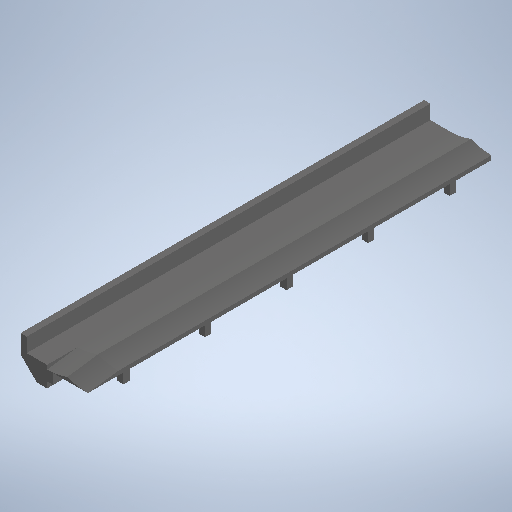
# Autodesk Inventor part: front_rail
Saved by Autodesk Inventor 2026.1 (Build 301233020, 233B)
## iProperties
Created: 2025-09-28
Part Number: front_rail
Material: 一般
Document SubType Name: Modeling
Designer: hibik
Density: 1 g/cm^3
Appearance: 既定
Author: hibik
Autodesk Inventor part; units mm, degrees
ref_plane "YZ Plane" through (0, 0, 0) normal (1, 0, 0) x (0, 1, 0)
ref_plane "XZ Plane" through (0, 0, 0) normal (0, 1, 0) x (-1, 0, 0)
ref_plane "XY Plane" through (0, 0, 0) normal (0, 0, 1) x (1, 0, 0)
sketch "スケッチ1" plane through (0, 0, 0) normal (0, 1, 0) x (-1, 0, 0)
  line L0 (0, 99) -> (20, 99)
  line L1 (20, 99) -> (20, -99)
  line L2 (20, -99) -> (0, -99)
  line L3 (0, -99) -> (0, 99)
  line L4 (20, -99) -> (20, -109)
  line L5 (20, -109) -> (9, -109)
  line L6 (9, -109) -> (11, -99)
  line L7 (10.5, 99) -> (8.5, 88.5)
  line L8 (8.5, 88.5) -> (20, 88.5)
  point P0 (0, 0)
  point P1 (0, 0)
  point P2 (10, -99)
  point P3 (10, 99)
  dimension "d0" = 198
  dimension "d1" = 20
  dimension "d4" = 10
  dimension "d5" = 1
  dimension "d6" = 1
  dimension "d7" = 10.5
  dimension "d8" = 1.5
  dimension "d9" = 0.5
  constraints: 18 end point, 3 midpoint, 3 perpendicular, 3 point on line, 2 parallel, 1 coincident, 1 horizontal, 1 vertical
  measures "d0" distance of L0.end L1.end
  measures "d1" distance of L0.start L0.end
  measures "d4" distance of L1.end L4.end
  measures "d5" distance of point (10, -99) L6.end
  measures "d6" horizontal distance of point (10, -99) L5.end
  measures "d7" distance between parallel lines of L0 L8
  measures "d8" horizontal distance of point (10, 99) L7.end
  measures "d9" distance of point (10, 99) L7.start
extrude "押し出し1" add sketch "スケッチ1" along normal blind 5.5 contours L0 L7 L8 L1 L2 L3 | L2 L4 L5 L6
sketch "スケッチ2" plane through (0, 5.5, 0) normal (0, 1, 0) x (1, 0, 0)
  line L0 (-20, 109) -> (-20, -88.5) projected
  line L1 (-20, -1.5) -> (-17, -1.5)
  line L2 (-17, -1.5) -> (-17, 1.5)
  line L3 (-17, 1.5) -> (-20, 1.5)
  line L4 (-20, 1.5) -> (-20, -1.5)
  line L5 (0, -99) -> (0, 99) projected
  line L6 (0, -1.5) -> (-3, -1.5)
  line L7 (-3, -1.5) -> (-3, 1.5)
  line L8 (-3, 1.5) -> (0, 1.5)
  line L9 (0, 1.5) -> (0, -1.5)
  point P0 (0, 0)
  point P1 (-17, 0)
  point P2 (0, 0)
  point P3 (0, 1.5)
  dimension "d10" = 3
  dimension "d11" = 3
  constraints: 16 end point, 4 parallel, 4 point on line, 2 horizontal, 2 midpoint, 2 perpendicular, 1 collinear, 1 horizontal alignment
  measures "d10" distance of L1.start L1.end
  measures "d11" distance of L1.end L2.end
extrude "押し出し2" cut sketch "スケッチ2" against normal through all
pattern_linear "矩形状パターン1" count 3 spacing 40 along (0, 0, -1) count 3 spacing 40 along (0, 0, 1) of "押し出し2"
sketch "スケッチ3" plane through (0, 5.5, 0) normal (0, 1, 0) x (1, 0, 0)
  line L0 (-20, -88.5) -> (-8.5, -88.5) projected
  line L1 (-20, -99) -> (0, -99)
  line L2 (0, -99) -> (0, 99)
  line L3 (0, 99) -> (-20.1365, 99)
  line L4 (-20, 109) -> (-20, -88.4991)
  line L5 (-20, -38.5) -> (-17, -38.5) projected
  line L6 (-17, -38.5) -> (-17, -41.5) projected
  line L7 (-17, -41.5) -> (-20, -41.5) projected
  line L8 (-20, -41.5) -> (-20, -78.5) projected
  line L9 (-20, -78.5) -> (-17, -78.5) projected
  line L10 (-17, -78.5) -> (-17, -81.5) projected
  line L11 (-17, -81.5) -> (-20, -81.5) projected
  line L12 (-20, -81.5) -> (-20, -88.5) projected
  line L13 (-20, -88.5) -> (-8.5, -88.5) projected
  line L14 (-8.5, -88.5) -> (-10.5, -99) projected
  line L15 (-10.5, -99) -> (0, -99) projected
  line L16 (0, -99) -> (0, -81.5) projected
  line L17 (0, -81.5) -> (-3, -81.5) projected
  line L18 (-3, -81.5) -> (-3, -78.5) projected
  line L19 (-3, -78.5) -> (0, -78.5) projected
  line L20 (0, -78.5) -> (0, -41.5) projected
  line L21 (0, -41.5) -> (-3, -41.5) projected
  line L22 (-3, -41.5) -> (-3, -38.5) projected
  line L23 (-3, -38.5) -> (0, -38.5) projected
  line L24 (0, -38.5) -> (0, -1.5) projected
  line L25 (0, -1.5) -> (-3, -1.5) projected
  line L26 (-3, -1.5) -> (-3, 1.5) projected
  line L27 (-3, 1.5) -> (0, 1.5) projected
  line L28 (0, 1.5) -> (0, 38.5) projected
  line L29 (0, 38.5) -> (-3, 38.5) projected
  line L30 (-3, 38.5) -> (-3, 41.5) projected
  line L31 (-3, 41.5) -> (0, 41.5) projected
  line L32 (0, 41.5) -> (0, 78.5) projected
  line L33 (0, 78.5) -> (-3, 78.5) projected
  line L34 (-3, 78.5) -> (-3, 81.5) projected
  line L35 (-3, 81.5) -> (0, 81.5) projected
  line L36 (0, 81.5) -> (0, 99) projected
  line L37 (0, 99) -> (-11, 99) projected
  line L38 (-11, 99) -> (-9, 109) projected
  line L39 (-9, 109) -> (-20, 109) projected
  line L40 (-20, 109) -> (-20, 81.5) projected
  line L41 (-20, 81.5) -> (-17, 81.5) projected
  line L42 (-17, 81.5) -> (-17, 78.5) projected
  line L43 (-17, 78.5) -> (-20, 78.5) projected
  line L44 (-20, 78.5) -> (-20, 41.5) projected
  line L45 (-20, 41.5) -> (-17, 41.5) projected
  line L46 (-17, 41.5) -> (-17, 38.5) projected
  line L47 (-17, 38.5) -> (-20, 38.5) projected
  line L48 (-20, 38.5) -> (-20, 1.5) projected
  line L49 (-20, 1.5) -> (-17, 1.5) projected
  line L50 (-17, 1.5) -> (-17, -1.5) projected
  line L51 (-17, -1.5) -> (-20, -1.5) projected
  line L52 (-20, -1.5) -> (-20, -38.5) projected
  line L53 (-20, 109) -> (-20, 81.5) projected
  line L54 (-20, -99) -> (-20, -88.4991)
  point P0 (0, 0)
  point P1 (-20, 99)
  point P2 (0, -78.5)
  point P3 (0, -38.5)
  point P4 (0, 41.5)
  point P5 (0, 81.5)
  point P6 (-10.5558, 101.2209)
  point P7 (-20, -88.4991)
  constraints: 10 end point, 5 point on line, 2 parallel, 1 horizontal, 1 perpendicular, 1 vertical
extrude "押し出し3" cut sketch "スケッチ3" against normal through all contours L4 L11 L10 L9 L7 L6 L5 L51 L50 L49 L47 L46 L45 L43 L42 L41 L3 L2 L35 L34 L33 L31 L30 L29 L27 L26 L25 L23 L22 L21 L19 L18 L17 L1 L14 L0 | L4 L39 L38 L3
extrude "押し出し4" add sketch "スケッチ3" against normal blind 5 contours L4 L9 L10 L11 | L4 L5 L6 L7 | L17 L18 L19 L2 | L4 L49 L50 L51 | L21 L22 L23 L2 | L4 L45 L46 L47 | L25 L26 L27 L2 | L4 L41 L42 L43 | L29 L30 L31 L2 | L33 L34 L35 L2
extrude "押し出し5" add sketch "スケッチ3" along normal blind 2 contours L4 L11 L10 L9 L7 L6 L5 L51 L50 L49 L47 L46 L45 L43 L42 L41 L3 L2 L35 L34 L33 L31 L30 L29 L27 L26 L25 L23 L22 L21 L19 L18 L17 L1 L14 L0 | L0 L14 L1 L54 | L4 L9 L10 L11 | L4 L5 L6 L7 | L17 L18 L19 L2 | L4 L49 L50 L51 | L21 L22 L23 L2 | L4 L45 L46 L47 | L25 L26 L27 L2 | L4 L41 L42 L43 | L29 L30 L31 L2 | L33 L34 L35 L2
sketch "スケッチ4" plane through (-20, 5.5, 99) normal (0, 0, 1) x (1, 0, 0)
  arc A0 (0, 2) -> (10, 4) centre (0, 28) ccw
  line L0 (0, 2) -> (20, 2) projected
  arc A1 (10, 4) -> (20, 2) centre (20, 28) ccw
  line L1 (10, 4) -> (10, 2) construction
  point P0 (20, -5.5)
  point P1 (14.6904, 2)
  point P2 (5.3096, 2)
  dimension "d27" = 2
  constraints: 4 point on circle, 2 centre point, 2 end point, 1 midpoint, 1 perpendicular, 1 tangent, 1 other
  measures "d27" distance of L1.start L1.end
extrude "押し出し6" add sketch "スケッチ4" against normal up to surface (198 mm away)
chamfer "面取り1" distance 2 distance2 15 2 edges at (-5.099, 8.0049, 99) (-14.901, 8.0049, 99) measured on face at (-5.1971, 7.5146, 99) measured on face at (-14.8029, 7.5146, 99)
sketch "スケッチ5" plane through (-20, 0.5, 81.5) normal (0, 0, 1) x (1, 0, 0)
  line L0 (-13, 14) -> (-10, 14)
  line L1 (-10, 14) -> (-10, -3)
  line L2 (-10, -3) -> (-13, -3)
  line L3 (-13, -3) -> (-13, 14)
  line L4 (-10, 7) -> (0, 7)
  line L5 (0, 7) -> (0, -3)
  line L6 (0, -3) -> (-10, -3)
  line L7 (-10, -3) -> (-10, 7)
  line L8 (0, -3) -> (140, -3) projected
  point P0 (20, -0.5)
  dimension "d33" = 10
  dimension "d34" = 3
  dimension "d35" = 7
  dimension "d38" = 10
  constraints: 16 end point, 4 parallel, 4 point on line, 2 horizontal, 2 perpendicular
  measures "d33" distance of L5.end L6.end
  measures "d34" distance of L1.end L2.end
  measures "d35" distance between parallel lines of L0 L4
  measures "d38" distance of L4.end L5.end
extrude "押し出し7" add sketch "スケッチ5" against normal up to surface (180.5 mm away)
chamfer "面取り2" distance 8 angle 45 1 edges at (-33, -2.5, -8.75)
sketch "スケッチ7" plane through (-20, 5.5, 81.5) normal (0, 0, 1) x (1, 0, 0)
  line L0 (-5, -8) -> (-13, 0) projected
  line L1 (-5, -8) -> (0, -8) projected
  line L2 (0, -8) -> (0, -5) projected
  line L3 (3, -5) -> (0, -5) projected
  line L4 (3, 0) -> (3, -5) projected
  line L5 (0, 0) -> (3, 0) projected
  line L6 (0, 2) -> (0, 0) projected
  line L7 (0, 2) -> (-10, 2) projected
  line L8 (-10, 2) -> (-10, 9) projected
  line L9 (-10, 9) -> (-13, 9) projected
  line L10 (-13, 9) -> (-13, 0) projected
  point P0 (20, -5.5)
extrude "押し出し8" add sketch "スケッチ7" along normal up to surface (17.5 mm away)
